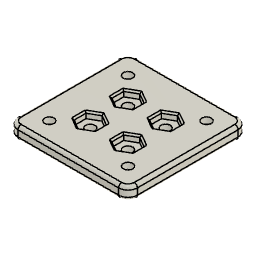
Foot_PartA_x6 (Autodesk Fusion 360 design; units mm, degrees)
Autodesk Fusion 360 part; units mm, degrees
sketch "Sketch1" plane through (0, 0, 0) normal (0, 0, 1) x (1, 0, 0)
  line L0 (0, 0) -> (34, 0)
  line L1 (34, 0) -> (34, 34)
  line L2 (34, 34) -> (0, 34)
  line L3 (0, 34) -> (0, 0)
  dimension "d1" = 34
  dimension "d2" = 34
  constraint horizontal L0
  constraint vertical L1
  constraint horizontal L2
  constraint vertical L3
  constraint coincident L0.start L3.end
  measures "d1" distance of L0.start L0.end
  measures "d2" distance of L0.start L2.end
extrude "Extrude1" add sketch "Sketch1" along normal blind 4
sketch "Sketch2" plane through (0, 0, 4) normal (0, 0, 1) x (-1, 0, 0)
  line L0 (0, -34) -> (0, 0)
  line L1 (0, 0) -> (-34, 0)
  line L2 (-34, 0) -> (-34, -34)
  line L3 (-34, -34) -> (0, -34)
  circle A0 centre (-4.5, -29.5) radius 1.5
  circle A1 centre (-29.5, -29.5) radius 1.5
  circle A2 centre (-29.5, -4.5) radius 1.5
  circle A3 centre (-4.5, -4.5) radius 1.5
  dimension "d8" = 3
  dimension "d9" = 3
  dimension "d10" = 3
  dimension "d11" = 3
  measures "d8" diameter of A0
  measures "d9" diameter of A1
  measures "d10" diameter of A2
  measures "d11" diameter of A3
extrude "Extrude3" cut sketch "Sketch2" against normal blind 9 contours A0 | A1 | A2 | A3
sketch "Sketch3" plane through (0, 0, 0) normal (0, 0, -1) x (1, 0, 0)
  circle A0 centre (29.5, -29.5) radius 1.5
  circle A1 centre (29.5, -4.5) radius 1.5
  circle A2 centre (4.5, -29.5) radius 1.5
  circle A3 centre (4.5, -4.5) radius 1.5
  line L0 (0, 0) -> (0, -34)
  line L1 (0, -34) -> (34, -34)
  line L2 (34, -34) -> (34, 0)
  line L3 (34, 0) -> (0, 0)
  line L4 (7.75, -2.6236) -> (4.5, -0.7472)
  line L5 (4.5, -0.7472) -> (1.25, -2.6236)
  line L6 (1.25, -2.6236) -> (1.25, -6.3764)
  line L7 (1.25, -6.3764) -> (4.5, -8.2528)
  line L8 (4.5, -8.2528) -> (7.75, -6.3764)
  line L9 (7.75, -6.3764) -> (7.75, -2.6236)
  line L10 (32.75, -2.6236) -> (29.5, -0.7472)
  line L11 (29.5, -0.7472) -> (26.25, -2.6236)
  line L12 (26.25, -2.6236) -> (26.25, -6.3764)
  line L13 (26.25, -6.3764) -> (29.5, -8.2528)
  line L14 (29.5, -8.2528) -> (32.75, -6.3764)
  line L15 (32.75, -6.3764) -> (32.75, -2.6236)
  line L16 (7.75, -27.6236) -> (4.5, -25.7472)
  line L17 (4.5, -25.7472) -> (1.25, -27.6236)
  line L18 (1.25, -27.6236) -> (1.25, -31.3764)
  line L19 (1.25, -31.3764) -> (4.5, -33.2528)
  line L20 (4.5, -33.2528) -> (7.75, -31.3764)
  line L21 (7.75, -31.3764) -> (7.75, -27.6236)
  line L22 (32.75, -27.6236) -> (29.5, -25.7472)
  line L23 (29.5, -25.7472) -> (26.25, -27.6236)
  line L24 (26.25, -27.6236) -> (26.25, -31.3764)
  line L25 (26.25, -31.3764) -> (29.5, -33.2528)
  line L26 (29.5, -33.2528) -> (32.75, -31.3764)
  line L27 (32.75, -31.3764) -> (32.75, -27.6236)
  point P0 (4.5, -4.5)
  point P1 (29.5, -4.5)
  point P2 (4.5, -29.5)
  point P3 (29.5, -29.5)
  dimension "d14" = 3.25
  dimension "d15" = 3.25
  dimension "d16" = 3.25
  dimension "d17" = 3.25
  constraint coincident P0 A3.centre
  constraint coincident P1 A1.centre
  constraint coincident P2 A2.centre
  constraint coincident P3 A0.centre
  measures "d14" distance of P0 L9
  measures "d15" distance of P1 L15
  measures "d16" distance of P2 L21
  measures "d17" distance of P3 L27
extrude "Extrude4" cut sketch "Sketch3" against normal blind 2 contours L4 L5 L6 L7 L8 L9 | L10 L11 L12 L13 L14 L15 | L16 L17 L18 L19 L20 L21 | L22 L23 L24 L25 L26 L27
chamfer "Chamfer2" distance 0.5 angle 45 24 edges at (31.125, 1.6854, 0) (27.875, 1.6854, 0) (26.25, 4.5, 0) (27.875, 7.3146, 0) (31.125, 7.3146, 0) (32.75, 4.5, 0) (6.125, 7.3146, 0) (2.875, 7.3146, 0) (1.25, 4.5, 0) (2.875, 1.6854, 0) (6.125, 1.6854, 0) (7.75, 4.5, 0) (6.125, 32.3146, 0) (7.75, 29.5, 0) (6.125, 26.6854, 0) (2.875, 26.6854, 0) (1.25, 29.5, 0) (2.875, 32.3146, 0) (27.875, 26.6854, 0) (31.125, 26.6854, 0) (32.75, 29.5, 0) (31.125, 32.3146, 0) (27.875, 32.3146, 0) (26.25, 29.5, 0)
extrude "Extrude5" add 1 faces at (22.6667, 34, 1.3333) along direction (0, 1, 0) blind 2
extrude "Extrude6" add 1 faces at (11.3333, 0, 1.3333) along direction (0, -1, 0) blind 2
extrude "Extrude7" add 1 faces at (34, 10.6667, 2.6667) along direction (1, 0, 0) blind 2
extrude "Extrude8" add 1 faces at (0, 10.6667, 2.6667) along direction (-1, 0, 0) blind 2
fillet "Fillet1" radius 3 4 edges at (36, 36, 2) (-2, 36, 2) (36, -2, 2) (-2, -2, 2)
fillet "Fillet2" radius 1 16 edges at (-2, 17, 0) (-1.1213, -1.1213, 0) (17, -2, 0) (35.1213, -1.1213, 0) (36, 17, 0) (35.1213, 35.1213, 0) (17, 36, 0) (-1.1213, 35.1213, 0) (17, -2, 4) (-1.1213, -1.1213, 4) (-2, 17, 4) (-1.1213, 35.1213, 4) (17, 36, 4) (35.1213, 35.1213, 4) (36, 17, 4) (35.1213, -1.1213, 4)
sketch "Sketch7" plane through (0, 0, 4) normal (0, 0, 1) x (-1, 0, 0)
  circle A0 centre (-29.5, -29.5) radius 1.5
  circle A1 centre (-29.5, -4.5) radius 1.5
  circle A2 centre (-4.5, -29.5) radius 1.5
  circle A3 centre (-4.5, -4.5) radius 1.5
  circle A4 centre (-11, -23) radius 1.5
  circle A5 centre (-23, -23) radius 1.5
  circle A6 centre (-11, -11) radius 1.5
  circle A7 centre (-23, -11) radius 1.5
  line L0 (-1, 1) -> (-33, 1)
  arc A8 (-33, 1) -> (-35, -1) centre (-33, -1) ccw
  line L1 (-35, -1) -> (-35, -33)
  arc A9 (-35, -33) -> (-33, -35) centre (-33, -33) ccw
  line L2 (-33, -35) -> (-1, -35)
  arc A10 (-1, -35) -> (1, -33) centre (-1, -33) ccw
  line L3 (1, -33) -> (1, -1)
  arc A11 (1, -1) -> (-1, 1) centre (-1, -1) ccw
  dimension "d40" = 3
  dimension "d41" = 3
  dimension "d42" = 3
  dimension "d43" = 3
  measures "d40" diameter of A4
  measures "d41" diameter of A5
  measures "d42" diameter of A6
  measures "d43" diameter of A7
extrude "Extrude11" cut sketch "Sketch7" against normal blind 5 contours A4 | A5 | A6 | A7
sketch "Sketch8" plane through (0, 0, 4) normal (0, 0, 1) x (-1, 0, 0)
  circle A0 centre (-11, -23) radius 1.5
  circle A1 centre (-11, -11) radius 1.5
  circle A2 centre (-23, -23) radius 1.5
  circle A3 centre (-23, -11) radius 1.5
  circle A4 centre (-29.5, -29.5) radius 1.5
  circle A5 centre (-29.5, -4.5) radius 1.5
  circle A6 centre (-4.5, -29.5) radius 1.5
  circle A7 centre (-4.5, -4.5) radius 1.5
  line L0 (-14.25, -24.8764) -> (-11, -26.7528)
  line L1 (-11, -26.7528) -> (-7.75, -24.8764)
  line L2 (-7.75, -24.8764) -> (-7.75, -21.1236)
  line L3 (-7.75, -21.1236) -> (-11, -19.2472)
  line L4 (-11, -19.2472) -> (-14.25, -21.1236)
  line L5 (-14.25, -21.1236) -> (-14.25, -24.8764)
  line L6 (-26.25, -24.8764) -> (-23, -26.7528)
  line L7 (-23, -26.7528) -> (-19.75, -24.8764)
  line L8 (-19.75, -24.8764) -> (-19.75, -21.1236)
  line L9 (-19.75, -21.1236) -> (-23, -19.2472)
  line L10 (-23, -19.2472) -> (-26.25, -21.1236)
  line L11 (-26.25, -21.1236) -> (-26.25, -24.8764)
  line L12 (-14.25, -12.8764) -> (-11, -14.7528)
  line L13 (-11, -14.7528) -> (-7.75, -12.8764)
  line L14 (-7.75, -12.8764) -> (-7.75, -9.1236)
  line L15 (-7.75, -9.1236) -> (-11, -7.2472)
  line L16 (-11, -7.2472) -> (-14.25, -9.1236)
  line L17 (-14.25, -9.1236) -> (-14.25, -12.8764)
  line L18 (-26.25, -12.8764) -> (-23, -14.7528)
  line L19 (-23, -14.7528) -> (-19.75, -12.8764)
  line L20 (-19.75, -12.8764) -> (-19.75, -9.1236)
  line L21 (-19.75, -9.1236) -> (-23, -7.2472)
  line L22 (-23, -7.2472) -> (-26.25, -9.1236)
  line L23 (-26.25, -9.1236) -> (-26.25, -12.8764)
  line L24 (-1, 1) -> (-33, 1)
  arc A8 (-33, 1) -> (-35, -1) centre (-33, -1) ccw
  line L25 (-35, -1) -> (-35, -33)
  arc A9 (-35, -33) -> (-33, -35) centre (-33, -33) ccw
  line L26 (-33, -35) -> (-1, -35)
  arc A10 (-1, -35) -> (1, -33) centre (-1, -33) ccw
  line L27 (1, -33) -> (1, -1)
  arc A11 (1, -1) -> (-1, 1) centre (-1, -1) ccw
  point P0 (-11, -23)
  point P1 (-23, -23)
  point P2 (-11, -11)
  point P3 (-23, -11)
  dimension "d46" = 3.25
  dimension "d49" = 3.25
  dimension "d50" = 3.25
  dimension "d51" = 3.25
  constraint coincident P0 A0.centre
  constraint coincident P1 A2.centre
  constraint coincident A1.centre P2
  constraint coincident P3 A3.centre
  measures "d46" distance of P0 L5
  measures "d49" distance of P1 L11
  measures "d50" distance of P2 L17
  measures "d51" distance of P3 L23
extrude "Extrude12" cut sketch "Sketch8" against normal blind 2 contours L0 L1 L2 L3 L4 L5 | L6 L7 L8 L9 L10 L11 | L12 L13 L14 L15 L16 L17 | L18 L19 L20 L21 L22 L23
chamfer "Chamfer3" distance 0.5 angle 45 24 edges at (12.625, 20.1854, 4) (14.25, 23, 4) (12.625, 25.8146, 4) (9.375, 25.8146, 4) (7.75, 23, 4) (9.375, 20.1854, 4) (21.375, 20.1854, 4) (24.625, 20.1854, 4) (26.25, 23, 4) (24.625, 25.8146, 4) (21.375, 25.8146, 4) (19.75, 23, 4) (9.375, 8.1854, 4) (12.625, 8.1854, 4) (14.25, 11, 4) (12.625, 13.8146, 4) (9.375, 13.8146, 4) (7.75, 11, 4) (21.375, 8.1854, 4) (24.625, 8.1854, 4) (26.25, 11, 4) (24.625, 13.8146, 4) (21.375, 13.8146, 4) (19.75, 11, 4)
